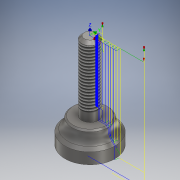
# Autodesk Inventor part: maniplo
Saved by Autodesk Inventor 2018 (Build 220112000, 112)
## iProperties
Created: 2018-05-11
Part Number: maniplo
Material: Aço, carbono
Document SubType Name: Modeling
Designer: Georgines
Density: 7.85 g/cm^3
Appearance: Semipolido
Author: Georgines
Autodesk Inventor part; units mm, degrees
ref_plane "YZ Plane" through (0, 0, 0) normal (1, 0, 0) x (0, 1, 0)
ref_plane "XZ Plane" through (0, 0, 0) normal (0, 1, 0) x (-1, 0, 0)
ref_plane "XY Plane" through (0, 0, 0) normal (0, 0, 1) x (1, 0, 0)
sketch "Esboço2" plane through (0, 0, 0) normal (0, 0, 1) x (1, 0, 0)
  circle A0 centre (0, 0) radius 9
  dimension "d10" = 18
  constraints: 1 centre point, 1 coincident
  measures "d10" diameter of A0
extrude "Extrusão1" add sketch "Esboço2" along normal blind 5
sketch "Esboço3" plane through (0, 0, 5) normal (0, 0, 1) x (1, 0, 0)
  circle A0 centre (0, 0) radius 6.5
  dimension "d13" = 13
  constraints: 1 centre point, 1 coincident
  measures "d13" diameter of A0
extrude "Extrusão2" add sketch "Esboço3" along normal blind 4
sketch "Esboço4" plane through (0, 0, 9) normal (0, 0, 1) x (1, 0, 0)
  circle A0 centre (0, 0) radius 3
  dimension "d17" = 6
  constraints: 1 centre point, 1 coincident
  measures "d17" diameter of A0
extrude "Extrusão3" add sketch "Esboço4" along normal blind 25
chamfer "Chanfro2" distance 1 angle 45 1 edges at (-3, 0, 34)
chamfer "Chanfro3" distance 0.5 angle 45 1 edges at (-6.5, 0, 9)
thread "Rosca1" size "M6x1" class "6g" standard "ISO Metric profile" length 25 offset 3
chamfer "Chanfro5" distance 1 angle 45 1 edges at (-9, 0, 5)
fillet "Arredondamento1" radius 5 1 edges at (-6.5, 0, 5)
